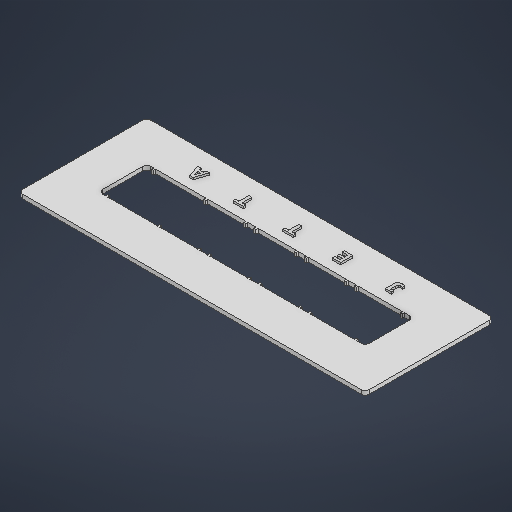
# Autodesk Inventor part: Plantilla_Jetta
Saved by Autodesk Inventor 2026.2 (Build 302298000, 298)
## iProperties
Created: 2026-03-21
Part Number: Plantilla_Jetta
Material: Generic
Document SubType Name: Modeling
Designer: Alejandro Rodriguez
Density: 1 g/cm^3
Appearance: Default
Author: Alejandro Rodriguez
Autodesk Inventor part; units mm, degrees
ref_plane "YZ Plane" through (0, 0, 0) normal (1, 0, 0) x (0, 1, 0)
ref_plane "XZ Plane" through (0, 0, 0) normal (0, 1, 0) x (-1, 0, 0)
ref_plane "XY Plane" through (0, 0, 0) normal (0, 0, 1) x (1, 0, 0)
sketch "Sketch1" plane through (0, 0, 0) normal (0, 1, 0) x (-1, 0, 0)
  line L0 (-66.5, 12) -> (66.5, 12)
  line L1 (66.5, 12) -> (66.5, -12)
  line L2 (66.5, -12) -> (-66.5, -12)
  line L3 (-66.5, -12) -> (-66.5, 12)
  line L4 (86.5, 32) -> (-86.5, 32)
  line L5 (-86.5, 32) -> (-86.5, -32)
  line L6 (-86.5, -32) -> (86.5, -32)
  line L7 (86.5, -32) -> (86.5, 32)
  line L8 (-62, -12) -> (-61, -12)
  line L9 (-61, -12) -> (-61, -11)
  line L10 (-61, -11) -> (-62, -11)
  line L11 (-62, -11) -> (-62, -12)
  line L12 (-39, -12) -> (-38, -12)
  line L13 (-38, -12) -> (-38, -11)
  line L14 (-38, -11) -> (-39, -11)
  line L15 (-39, -11) -> (-39, -12)
  line L16 (-33, -12) -> (-33, -11)
  line L17 (-34, -12) -> (-33, -12)
  line L18 (-33, -11) -> (-34, -11)
  line L19 (-34, -11) -> (-34, -12)
  line L20 (-14, -11) -> (-14, -12)
  line L21 (-13, -12) -> (-13, -11)
  line L22 (-14, -12) -> (-13, -12)
  line L23 (-13, -11) -> (-14, -11)
  line L24 (-8, -11) -> (-9, -11)
  line L25 (-8, -12) -> (-8, -11)
  line L26 (-9, -11) -> (-9, -12)
  line L27 (-9, -12) -> (-8, -12)
  line L28 (11, -12) -> (12, -12)
  line L29 (12, -12) -> (12, -11)
  line L30 (12, -11) -> (11, -11)
  line L31 (11, -11) -> (11, -12)
  line L32 (17, -11) -> (16, -11)
  line L33 (16, -11) -> (16, -12)
  line L34 (16, -12) -> (17, -12)
  line L35 (17, -12) -> (17, -11)
  line L36 (36, -11) -> (36, -12)
  line L37 (37, -11) -> (36, -11)
  line L38 (37, -12) -> (37, -11)
  line L39 (36, -12) -> (37, -12)
  line L40 (62, -11) -> (62, -12)
  line L41 (63, -12) -> (63, -11)
  line L42 (63, -11) -> (62, -11)
  line L43 (62, -12) -> (63, -12)
  line L44 (-66.5, 0) -> (66.5, 0) construction
  line L45 (-62, 12) -> (-61, 12)
  line L46 (-61, 12) -> (-61, 11)
  line L47 (-61, 11) -> (-62, 11)
  line L48 (-62, 11) -> (-62, 12)
  line L49 (-38, 12) -> (-38, 11)
  line L50 (-39, 12) -> (-38, 12)
  line L51 (-38, 11) -> (-39, 11)
  line L52 (-39, 11) -> (-39, 12)
  line L53 (-34, 11) -> (-34, 12)
  line L54 (-33, 12) -> (-33, 11)
  line L55 (-34, 12) -> (-33, 12)
  line L56 (-33, 11) -> (-34, 11)
  line L57 (-13, 11) -> (-14, 11)
  line L58 (-13, 12) -> (-13, 11)
  line L59 (-14, 11) -> (-14, 12)
  line L60 (-14, 12) -> (-13, 12)
  line L61 (-9, 12) -> (-8, 12)
  line L62 (-8, 12) -> (-8, 11)
  line L63 (-8, 11) -> (-9, 11)
  line L64 (-9, 11) -> (-9, 12)
  line L65 (12, 11) -> (11, 11)
  line L66 (11, 11) -> (11, 12)
  line L67 (11, 12) -> (12, 12)
  line L68 (12, 12) -> (12, 11)
  line L69 (16, 11) -> (16, 12)
  line L70 (17, 11) -> (16, 11)
  line L71 (17, 12) -> (17, 11)
  line L72 (16, 12) -> (17, 12)
  line L73 (36, 11) -> (36, 12)
  line L74 (37, 12) -> (37, 11)
  line L75 (37, 11) -> (36, 11)
  line L76 (36, 12) -> (37, 12)
  line L77 (62, 12) -> (63, 12)
  line L78 (62, 11) -> (62, 12)
  line L79 (63, 11) -> (62, 11)
  line L80 (63, 12) -> (63, 11)
  point P0 (0, 0)
  point P1 (0, 12)
  point P2 (-61.5, -12)
  point P3 (-61.5, -11)
  point P4 (-38.5, -12)
  point P5 (-38.5, -11)
  point P6 (-33.5, -12)
  point P7 (-33.5, -11)
  point P8 (-13.5, -11)
  point P9 (-13.5, -12)
  point P10 (-8.5, -11)
  point P11 (-8.5, -12)
  point P12 (11.5, -12)
  point P13 (11.5, -11)
  point P14 (16.5, -11)
  point P15 (16.5, -12)
  point P16 (36.5, -11)
  point P17 (36.5, -12)
  point P18 (62.5, -12)
  point P19 (62.5, -11)
  point P20 (-61.5, 12)
  point P21 (-61.5, 11)
  point P22 (-38.5, 12)
  point P23 (-38.5, 11)
  point P24 (-33.5, 11)
  point P25 (-33.5, 12)
  point P26 (-13.5, 11)
  point P27 (-13.5, 12)
  point P28 (-8.5, 12)
  point P29 (-8.5, 11)
  point P30 (11.5, 11)
  point P31 (11.5, 12)
  point P32 (16.5, 11)
  point P33 (16.5, 12)
  point P34 (36.5, 12)
  point P35 (36.5, 11)
  point P36 (62.5, 12)
  point P37 (62.5, 11)
  point P38 (63, -12)
  point P39 (62, -12)
  point P40 (37, -12)
  point P41 (36, -12)
  point P42 (17, -12)
  point P43 (16, -12)
  point P44 (12, -12)
  point P45 (11, -12)
  point P46 (-8, -12)
  point P47 (-9, -12)
  point P48 (-13, -12)
  point P49 (-14, -12)
  point P50 (-33, -12)
  point P51 (-34, -12)
  point P52 (-38, -12)
  point P53 (-39, -12)
  point P54 (-61, -12)
  point P55 (-62, -12)
  point P56 (-62, 12)
  point P57 (-61, 12)
  point P58 (-39, 12)
  point P59 (-38, 12)
  point P60 (-34, 12)
  point P61 (-33, 12)
  point P62 (-14, 12)
  point P63 (-13, 12)
  point P64 (-9, 12)
  point P65 (-8, 12)
  point P66 (11, 12)
  point P67 (12, 12)
  point P68 (16, 12)
  point P69 (17, 12)
  point P70 (36, 12)
  point P71 (37, 12)
  point P72 (62, 12)
  point P73 (63, 12)
  dimension "d0" = 133
  dimension "d1" = 24
  dimension "d2" = 20
  dimension "d3" = 1
  dimension "d4" = 1
  dimension "d5" = 5
  dimension "d6" = 1
  dimension "d7" = 1
  dimension "d8" = 23
  dimension "d9" = 1
  dimension "d10" = 1
  dimension "d11" = 5
  dimension "d12" = 1
  dimension "d13" = 1
  dimension "d14" = 20
  dimension "d15" = 1
  dimension "d16" = 1
  dimension "d17" = 5
  dimension "d18" = 1
  dimension "d19" = 1
  dimension "d20" = 20
  dimension "d21" = 1
  dimension "d22" = 1
  dimension "d23" = 5
  dimension "d24" = 1
  dimension "d25" = 1
  dimension "d26" = 20
  dimension "d27" = 1
  dimension "d28" = 1
  dimension "d29" = 26
  constraints: 158 end point, 54 symmetric about line, 21 parallel, 20 midpoint, 10 horizontal, 10 perpendicular, 1 horizontal alignment, 1 vertical, 1 vertical alignment, 19 other
  measures "d0" distance of L3.end L1.start
  measures "d1" distance of L3.start L3.end
  measures "d3" distance of L8.start L8.end
  measures "d4" distance of L10.end L8.start
  measures "d5" distance from line of L3 point (-61.5, -11)
  measures "d6" distance of L12.start L13.start
  measures "d7" distance of L14.end L12.start
  measures "d8" horizontal distance of point (-61.5, -11) point (-38.5, -12)
  measures "d9" distance of L19.end L16.start
  measures "d10" distance of L19.start L19.end
  measures "d11" distance of point (-33.5, -12) point (-38.5, -12)
  measures "d12" distance of L20.end L21.start
  measures "d13" distance of L23.end L20.end
  measures "d14" distance of point (-13.5, -12) point (-33.5, -12)
  measures "d15" distance of L27.start L27.end
  measures "d16" distance of L24.end L27.start
  measures "d17" distance of point (-8.5, -12) point (-13.5, -12)
  measures "d18" distance of L31.end L28.end
  measures "d19" distance of L30.end L31.end
  measures "d20" distance of point (-8.5, -12) point (11.5, -12)
  measures "d21" distance of L33.end L35.start
  measures "d22" distance of L33.start L33.end
  measures "d23" distance of point (16.5, -12) point (11.5, -12)
  measures "d24" distance of L36.end L38.start
  measures "d25" distance of L36.start L36.end
  measures "d26" distance of point (36.5, -12) point (16.5, -12)
  measures "d27" distance of L43.start L43.end
  measures "d28" distance of L40.start L43.start
  measures "d29" distance of point (62.5, -12) point (36.5, -12)
extrude "Extrusion1" add sketch "Sketch1" along normal blind 2 contours L0 L46 L47 L48 | L11 L10 L9 L2 | L0 L49 L51 L52 | L15 L14 L13 L2 | L0 L54 L56 L53 | L19 L18 L16 L2 | L0 L58 L57 L59 | L20 L23 L21 L2 | L0 L62 L63 L64 | L26 L24 L25 L2 | L0 L68 L65 L66 | L31 L30 L29 L2 | L0 L71 L70 L69 | L33 L32 L35 L2 | L0 L74 L75 L73 | L36 L37 L38 L2 | L0 L80 L79 L78 | L40 L42 L41 L2 | L7 L6 L5 L4
sketch "Sketch4" plane through (0, 0, 0) normal (0, 1, 0) x (-1, 0, 0)
  line L0 (-26.0735, -16.7591) -> (-15.6042, -16.7591) construction
  line L1 (-15.6042, -16.7591) -> (-15.6042, -26.2935) construction
  line L2 (-15.6042, -26.2935) -> (-26.0735, -26.2935) construction
  line L3 (-26.0735, -26.2935) -> (-26.0735, -16.7591) construction
  line L4 (-59.7082, -16.7591) -> (-80.6467, -17.2409) construction
  line L5 (-80.6467, -17.2409) -> (-80.4274, -26.7728) construction
  line L6 (-80.4274, -26.7728) -> (-59.4889, -26.2911) construction
  line L7 (-59.4889, -26.2911) -> (-59.7082, -16.7591) construction
  line L8 (-1.8321, -16.7591) -> (8.6372, -16.7591) construction
  line L9 (8.6372, -16.7591) -> (8.6372, -26.2935) construction
  line L10 (8.6372, -26.2935) -> (-1.8321, -26.2935) construction
  line L11 (-1.8321, -26.2935) -> (-1.8321, -16.7591) construction
  line L12 (46.0957, -26.2935) -> (46.0957, -16.7591) construction
  line L13 (46.0957, -16.7591) -> (56.565, -16.7591) construction
  line L14 (56.565, -16.7591) -> (56.565, -26.2935) construction
  line L15 (56.565, -26.2935) -> (46.0957, -26.2935) construction
  line L16 (20.4435, -23.6306) -> (20.4435, -14.4576) construction
  line L17 (20.4435, -14.4576) -> (30.9128, -14.4576) construction
  line L18 (30.9128, -14.4576) -> (30.9128, -23.6306) construction
  line L19 (30.9128, -23.6306) -> (20.4435, -23.6306) construction
  line L20 (23.0931, -25.9322) -> (23.0931, -16.7591) construction
  line L21 (23.0931, -16.7591) -> (33.5623, -16.7591) construction
  line L22 (33.5623, -16.7591) -> (33.5623, -25.9322) construction
  line L23 (33.5623, -25.9322) -> (23.0931, -25.9322) construction
  line L24 (-39, -12) -> (-61, -12) projected
  line L25 (-25.4412, -22.8551) -> (-25.4412, -16.7591)
  line L26 (-25.4412, -16.7591) -> (-21.3212, -16.7591)
  line L27 (-21.3212, -16.7591) -> (-21.3212, -17.92)
  line L28 (-21.3212, -17.92) -> (-23.9197, -17.92)
  line L29 (-23.9197, -17.92) -> (-23.9197, -18.992)
  line L30 (-23.9197, -18.992) -> (-21.5237, -18.992)
  line L31 (-21.5237, -18.992) -> (-21.5237, -20.1529)
  line L32 (-21.5237, -20.1529) -> (-23.9197, -20.1529)
  line L33 (-23.9197, -20.1529) -> (-23.9197, -21.6942)
  line L34 (-23.9197, -21.6942) -> (-21.3212, -21.6942)
  line L35 (-21.3212, -21.6942) -> (-21.3212, -22.8551)
  line L36 (-21.3212, -22.8551) -> (-25.4412, -22.8551)
  line L37 (-0.029, -22.8551) -> (-0.029, -17.92)
  line L38 (-0.029, -17.92) -> (-1.8321, -17.92)
  line L39 (-1.8321, -17.92) -> (-1.8321, -16.7591)
  line L40 (-1.8321, -16.7591) -> (3.3055, -16.7591)
  line L41 (3.3055, -16.7591) -> (3.3055, -17.92)
  line L42 (3.3055, -17.92) -> (1.5024, -17.92)
  line L43 (1.5024, -17.92) -> (1.5024, -22.8551)
  line L44 (1.5024, -22.8551) -> (-0.029, -22.8551)
  line L45 (24.8962, -22.8551) -> (24.8962, -17.92)
  line L46 (24.8962, -17.92) -> (23.0931, -17.92)
  line L47 (23.0931, -17.92) -> (23.0931, -16.7591)
  line L48 (23.0931, -16.7591) -> (28.2307, -16.7591)
  line L49 (28.2307, -16.7591) -> (28.2307, -17.92)
  line L50 (28.2307, -17.92) -> (26.4276, -17.92)
  line L51 (26.4276, -17.92) -> (26.4276, -22.8551)
  line L52 (26.4276, -22.8551) -> (24.8962, -22.8551)
  line L53 (46.071, -22.8551) -> (48.131, -16.7591)
  line L54 (48.131, -16.7591) -> (49.8008, -16.7591)
  line L55 (49.8008, -16.7591) -> (51.8608, -22.8551)
  line L56 (51.8608, -22.8551) -> (50.2849, -22.8551)
  line L57 (50.2849, -22.8551) -> (49.9045, -21.6102)
  line L58 (49.9045, -21.6102) -> (47.9878, -21.6102)
  line L59 (47.9878, -21.6102) -> (47.6025, -22.8551)
  line L60 (47.6025, -22.8551) -> (46.071, -22.8551)
  line L61 (49.5686, -20.5037) -> (48.9461, -18.4881)
  line L62 (48.9461, -18.4881) -> (48.3188, -20.5037)
  line L63 (48.3188, -20.5037) -> (49.5686, -20.5037)
  point P0 (0, 0)
  point P1 (-70.1775, -17)
  point P2 (3.4025, -16.7591)
  point P3 (28.3277, -16.7591)
  point P4 (51.3304, -16.7591)
  dimension "d34" = 5
  constraints: 4 horizontal alignment, 4 midpoint, 11 other
  measures "d34" distance from line of L24 point (-70.177, -17)
extrude "Extrusion2" add sketch "Sketch4" along normal blind 3
sketch "Sketch5" plane through (0, 0, 0) normal (0, 1, 0) x (-1, 0, 0)
  line L0 (-51.4817, -16.7591) -> (-43.9207, -16.7591) construction
  line L1 (-43.9207, -16.7591) -> (-43.9207, -23.2058) construction
  line L2 (-43.9207, -23.2058) -> (-51.4817, -23.2058) construction
  line L3 (-51.4817, -23.2058) -> (-51.4817, -16.7591) construction
  line L4 (-21.3212, -16.7591) -> (-25.4412, -16.7591) projected
  spline S0 degree 2 poles (-47.8409, -21.0668) (-47.8409, -21.462) (-48.1126, -22.1635) (-48.3843, -22.4105) knots 0 0 0 1 2 2 2
  spline S1 degree 2 poles (-48.3843, -22.4105) (-48.6906, -22.6872) (-49.5254, -22.949) (-50.0688, -22.949) knots 0 0 0 1 2 2 2
  spline S2 degree 2 poles (-50.0688, -22.949) (-50.4739, -22.949) (-51.1853, -22.8897) (-51.457, -22.8304) knots 0 0 0 1 2 2 2
  line L5 (-51.457, -22.8304) -> (-51.457, -21.5954)
  line L6 (-51.457, -21.5954) -> (-51.3187, -21.5954)
  spline S3 degree 2 poles (-51.3187, -21.5954) (-51.1359, -21.6695) (-50.7357, -21.798) (-50.4196, -21.798) knots 0 0 0 1 2 2 2
  spline S4 degree 2 poles (-50.4196, -21.798) (-50.0145, -21.798) (-49.5748, -21.5707) (-49.4859, -21.3632) knots 0 0 0 1 2 2 2
  spline S5 degree 2 poles (-49.4859, -21.3632) (-49.3921, -21.1607) (-49.3723, -20.6371) (-49.3723, -20.311) knots 0 0 0 1 2 2 2
  line L7 (-49.3723, -20.311) -> (-49.3723, -17.8657)
  line L8 (-49.3723, -17.8657) -> (-50.7654, -17.8657)
  line L9 (-50.7654, -17.8657) -> (-50.7654, -16.7591)
  line L10 (-50.7654, -16.7591) -> (-47.8409, -16.7591)
  line L11 (-47.8409, -16.7591) -> (-47.8409, -21.0668)
  point P0 (0, 0)
  point P1 (-47.7012, -16.7591)
  point P2 (-23.3812, -16.7591)
  constraints: 2 midpoint, 1 horizontal alignment, 2 other
extrude "Extrusion3" add sketch "Sketch5" along normal blind 3
fillet "Fillet1" radius 2 8 edges at (-86.5, 1, -32) (-86.5, 1, 32) (86.5, 1, 32) (86.5, 1, -32) (66.5, 1, 12) (66.5, 1, -12) (-66.5, 1, 12) (-66.5, 1, -12)
body "Solid1"
